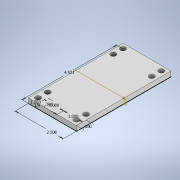
# Autodesk Inventor part: USAXS Rail Extender
Saved by Autodesk Inventor 2020 (Build 240168000, 168)
## iProperties
Created: 2022-06-25
Part Number: USAXS Rail Extender
Material: Generic
Document SubType Name: Modeling
Designer: Beaucage
Density: 1 g/cm^3
Appearance: Default
Author: Beaucage
Autodesk Inventor part; units mm, degrees
ref_plane "YZ Plane" through (0, 0, 0) normal (1, 0, 0) x (0, 1, 0)
ref_plane "XZ Plane" through (0, 0, 0) normal (0, 1, 0) x (-1, 0, 0)
ref_plane "XY Plane" through (0, 0, 0) normal (0, 0, 1) x (1, 0, 0)
sketch "Sketch1" plane through (0, 0, 0) normal (0, 1, 0) x (-1, 0, 0)
  line L0 (0, 0) -> (63.5, 0)
  line L1 (63.5, 0) -> (63.5, -125)
  line L2 (63.5, -125) -> (0, -125)
  line L3 (0, -125) -> (0, 0)
  line L4 (63.5, 0) -> (63.5, -6.35)
  line L5 (63.5, -6.35) -> (31.75, -6.35)
  line L6 (31.75, -6.35) -> (57.15, -6.35)
  line L7 (31.75, -6.35) -> (6.35, -6.35)
  line L8 (6.35, -6.35) -> (6.35, -19.05)
  line L9 (57.15, -6.35) -> (57.15, -19.05)
  dimension "d0" = 125
  dimension "d1" = 6.35
  dimension "d2" = 25.4
  dimension "d3" = 63.5
  dimension "d4" = 31.75
  dimension "d5" = 25.4
  dimension "d6" = 12.7
  dimension "d7" = 12.7
  constraints: 20 end point, 2 horizontal, 2 parallel, 2 perpendicular, 2 point on line, 2 vertical
  measures "d0" distance of L0.end L1.end
  measures "d1" distance of L0.end L4.end
  measures "d2" distance of L5.end L6.end
  measures "d3" distance between parallel lines of L3 L1
  measures "d4" distance of L4.end L5.end
  measures "d5" distance of L5.end L7.end
  measures "d6" distance of L7.end L8.end
  measures "d7" distance of L6.end L9.end
extrude "Extrusion1" add sketch "Sketch1" along normal blind 6.35
hole "Hole1" at (-6.35, 0, -6.35) at (-6.35, 0, -19.05) at (-57.15, 0, -6.35) at (-57.15, 0, -19.05) direction (0, 1, 0) diameter 6.7564 end through all clearance for "Socket Head Cap Screw" size "1/4" standard "Ansi Unified Screw Threads"
ref_plane "Work Plane1" through (0, 6.35, -62.5) normal (0, 0, 1) x (1, 0, 0)
mirror "Mirror1" about plane through (0, 6.35, -62.5) normal (0, 0, 1) of "Hole1"
body "Solid1"
